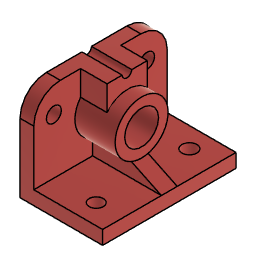
Exercise 5_ (Autodesk Fusion 360 design; units mm, degrees)
Autodesk Fusion 360 part; units mm, degrees
sketch "Sketch1" plane through (0, 0, 0) normal (0, 1, 0) x (1, 0, 0)
  line L0 (0, 0) -> (0, -90)
  line L1 (0, -90) -> (13, -90)
  line L2 (13, -90) -> (13, -13)
  line L3 (0, 0) -> (78, 0)
  line L4 (78, 0) -> (78, -13)
  line L5 (78, -13) -> (13, -13)
  dimension "d1" = 90
  dimension "d2" = 13
  dimension "d3" = 77
  dimension "d6" = 78
  constraint coincident L0.start L3.start
  constraint vertical L0
  constraint perpendicular L0 L1
  constraint perpendicular L1 L2
  constraint perpendicular L3 L4
  constraint perpendicular L2 L5
  measures "d1" distance of L0.start L0.end
  measures "d2" distance of L0.end L1.end
  measures "d3" distance of L1.end L2.end
  measures "d6" distance of L0.start L3.end
extrude "Extrude1" add sketch "Sketch1" along normal blind 126
sketch "Sketch2" plane through (0, 0, 13) normal (0, 0, 1) x (-1, 0, 0)
  line L0 (-13, 0) -> (-78, 0)
  line L1 (-78, 0) -> (-78, -126)
  line L2 (-78, -126) -> (-13, -126)
  line L3 (-13, -126) -> (-13, 0)
  circle A0 centre (-53, -107) radius 7.0711
  circle A1 centre (-53, -19) radius 6.6722
  dimension "d9" = 19
  dimension "d10" = 25
  dimension "d11" = 19
  dimension "d12" = 25
  measures "d9" distance of L2 A0.centre
  measures "d10" distance of L1 A0.centre
  measures "d11" distance of L0 A1.centre
  measures "d12" distance of L1 A1.centre
extrude "Extrude2" cut sketch "Sketch2" against normal blind 40 contours A0 | A1
sketch "Sketch3" plane through (13, 0, 0) normal (1, 0, 0) x (0, 1, 0)
  line L0 (0, 90) -> (0, 13)
  line L1 (0, 13) -> (126, 13)
  line L2 (126, 13) -> (126, 90)
  line L3 (126, 90) -> (0, 90)
  circle A0 centre (19, 65) radius 7.0711
  circle A1 centre (107, 65) radius 7.0711
  dimension "d15" = 25
  dimension "d16" = 19
  dimension "d17" = 25
  dimension "d18" = 19
  measures "d15" distance of L3 A0.centre
  measures "d16" distance of L0 A0.centre
  measures "d17" distance of L3 A1.centre
  measures "d18" distance of L2 A1.centre
extrude "Extrude3" cut sketch "Sketch3" against normal blind 110 contours A0 | A1
fillet "Fillet1" radius 25 2 edges at (6.5, 0, 90) (6.5, 126, 90)
sketch "Sketch4" plane through (13, 0, 0) normal (1, 0, 0) x (0, 1, 0)
  circle A0 centre (19, 65) radius 7.0711
  circle A1 centre (107, 65) radius 7.0711
  arc A2 (126, 65) -> (101, 90) centre (101, 65) ccw
  line L0 (101, 90) -> (25, 90)
  arc A3 (25, 90) -> (0, 65) centre (25, 65) ccw
  line L1 (0, 65) -> (0, 13)
  line L2 (0, 13) -> (126, 13)
  line L3 (126, 13) -> (126, 65)
  line L4 (19, 65) -> (107, 65) construction
  line L5 (82.2164, 65.1329) -> (44.2164, 65.1329)
  line L6 (44.2164, 65.1329) -> (44.2164, 90.1329)
  line L7 (44.2164, 90.1329) -> (82.2164, 90.1329)
  line L8 (82.2164, 90.1329) -> (82.2164, 65.1329)
  circle A4 centre (63, 90) radius 4.5
  point P0 (63.2164, 77.6329)
  dimension "d23" = 38
  dimension "d24" = 25
  dimension "d25" = 9
  constraint coincident A0.centre L4.start
  constraint coincident A1.centre L4.end
  constraint horizontal L5
  constraint perpendicular L5 L6
  constraint parallel L5 L7
  constraint parallel L6 L8
  constraint midpoint L0 A4.centre
  measures "d23" distance of L6.end L7.end
  measures "d24" distance of L5.end L6.end
  measures "d25" diameter of A4
extrude "Extrude4" cut sketch "Sketch4" against normal blind 32 contours L0 A4 | L7 A4
extrude "Extrude5" add sketch "Sketch4" along normal blind 25 contours L0 L5 L6 L8 A4
sketch "Sketch5" plane through (13, 0, 0) normal (1, 0, 0) x (0, 1, 0)
  line L0 (44.2164, 65.1329) -> (44.2164, 90)
  line L1 (44.2164, 90) -> (25, 90)
  arc A0 (25, 90) -> (0, 65) centre (25, 65) ccw
  line L2 (0, 65) -> (0, 13)
  line L3 (0, 13) -> (126, 13)
  line L4 (126, 13) -> (126, 65)
  arc A1 (126, 65) -> (101, 90) centre (101, 65) ccw
  line L5 (101, 90) -> (82.2164, 90)
  line L6 (82.2164, 90) -> (82.2164, 65.1329)
  line L7 (82.2164, 65.1329) -> (44.2164, 65.1329)
  circle A2 centre (19, 65) radius 7.0711
  circle A3 centre (107, 65) radius 7.0711
  circle A4 centre (63.8666, 51) radius 16
  circle A5 centre (63.8666, 51) radius 25
  dimension "d30" = 38
  dimension "d31" = 32
  dimension "d32" = 50
  constraint concentric A4 A5
  measures "d30" distance of L3 A4.centre
  measures "d31" diameter of A4
  measures "d32" diameter of A5
extrude "Extrude6" cut sketch "Sketch5" along normal blind 46 contours L0 L6 L7 A4 A5 | L0 L6 L7 A4 A5
delete_face "DeleteFace1" 1 faces at (29.6667, 70.0234, 65.768)
extrude "Extrude7" add sketch "Sketch5" along normal blind 38 contours L0 L6 L7 A4 A5 | L0 L6 L7 A4 A5
ref_plane "WorkPlane1" through (0, 63, 0) normal (0, 1, 0) x (0, 0, 1)
sketch "Sketch6" plane through (0, 63, 0) normal (0, 1, 0) x (1, 0, 0)
  line L0 (51, -26) -> (78, -13)
rib "Rib1" add thickness 15 on both sides direction (-0.433816, 0, -0.901002) up to next extending the curves path "Sketch6" along L0
